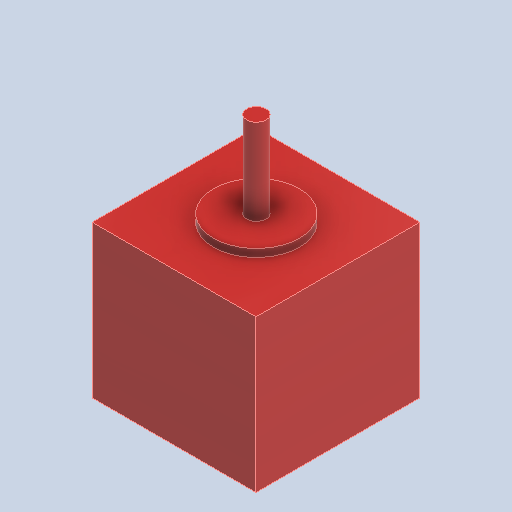
# Autodesk Inventor part: motor
Saved by Autodesk Inventor 2023 (Build 270158000, 158)
## iProperties
Created: 2024-08-03
Part Number: motor
Material: Generic
Document SubType Name: Modeling
Designer: sebas
Density: 1 g/cm^3
Appearance: Orange-Red
Mass: 69.9882 g
Surface Area: 105.638 cm^2
Volume: 69.9882 cm^3
Author: sebas
Autodesk Inventor part; units mm, degrees
ref_plane "YZ Plane" through (0, 0, 0) normal (1, 0, 0) x (0, 1, 0)
ref_plane "XZ Plane" through (0, 0, 0) normal (0, 1, 0) x (-1, 0, 0)
ref_plane "XY Plane" through (0, 0, 0) normal (0, 0, 1) x (1, 0, 0)
sketch "Sketch1" plane through (0, 0, 0) normal (0, 1, 0) x (-1, 0, 0)
  line L0 (0, 0) -> (0, -42)
  line L1 (0, -42) -> (42, -42)
  line L2 (42, -42) -> (42, 0)
  line L3 (42, 0) -> (0, 0)
  line L4 (0, 0) -> (42, 0)
  dimension "d0" = 42
  dimension "d1" = 42
  constraints: 10 end point, 4 perpendicular, 1 vertical
  measures "d0" distance of L0.start L0.end
  measures "d1" distance of L0.end L1.end
extrude "Extrusion1" add sketch "Sketch1" along normal blind 39
sketch "Sketch2" plane through (0, 39, 0) normal (0, 1, 0) x (1, 0, 0)
  line L0 (0, 0) -> (0, 42) projected
  line L1 (-41.7664, 0) -> (0, 42)
  circle A0 centre (-20.8832, 21) radius 11
  dimension "d4" = 22
  constraints: 2 end point, 1 centre point, 1 midpoint
  measures "d4" diameter of A0
extrude "Extrusion2" add sketch "Sketch2" along normal blind 2
sketch "Sketch3" plane through (-20.8832, 41, -21) normal (0, 1, 0) x (1, 0, 0)
  circle A0 centre (0, 0) radius 2.5
  point P0 (20.8832, -21)
  dimension "d7" = 5
  constraints: 1 centre point
  measures "d7" diameter of A0
extrude "Extrusion3" add sketch "Sketch3" along normal blind 22
body "Solid1"
